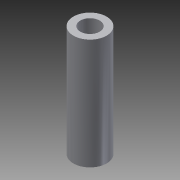
# Autodesk Inventor part: PS20002
Saved by Autodesk Inventor 2014 (Build 180170000, 170)
## iProperties
Category: Need To
Created: 2013-05-29
Part Number: PS20002
Material: Aluminum 6061
Document SubType Name: Modeling
Designer: Edward
Density: 2.71 g/cm^3
Catalog Web Link: http://aluminumspacers.com/
Description: 3/8" x 1-1/4" x #12 bore, aluminum spacer
Mass: 4.04 g
Surface Area: 15.9883 cm^2
Volume: 1.49077 cm^3
Stock Number: AS38-12-80
Vendor: aluminumspacers.com
Project: Shapeoko
Appearance: Aluminum - Flat
User Status: F
Authority: ALUMINUMSPACERS.COM, 8-2-13
Author: Edward
Subject: Spacers
Comments: Fusion
Autodesk Inventor part; units mm, degrees
ref_plane "YZ Plane" through (0, 0, 0) normal (1, 0, 0) x (0, 1, 0)
ref_plane "XZ Plane" through (0, 0, 0) normal (0, 1, 0) x (-1, 0, 0)
ref_plane "XY Plane" through (0, 0, 0) normal (0, 0, 1) x (1, 0, 0)
sketch "Sketch1" plane through (0, 0, 0) normal (0, 0, 1) x (1, 0, 0)
  circle A0 centre (0, 0) radius 4.7625
  circle A1 centre (0, 0) radius 2.7813
  dimension "d0" = 9.525
  dimension "d1" = 5.5626
  constraints: 2 centre point, 2 coincident
  measures "d0" diameter of A0
  measures "d1" diameter of A1
extrude "Extrusion1" add sketch "Sketch1" along normal blind 31.75
body "Solid1"
